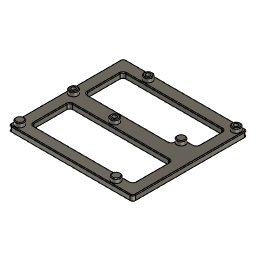
Manta-E3EZ_Mount (Autodesk Fusion 360 design; units mm, degrees)
Autodesk Fusion 360 part; units mm, degrees
sketch "Sketch1" plane through (0, 0, 0) normal (0, 0, 1) x (1, 0, 0)
  line L0 (0, 0) -> (120, 0)
  line L1 (120, 0) -> (120, 90.8)
  line L2 (120, 90.8) -> (0, 90.8)
  line L3 (0, 90.8) -> (0, 0)
  circle A0 centre (101.8, 77.23) radius 3
  circle A1 centre (39.65, 77.03) radius 3
  circle A2 centre (21.79, 42.05) radius 3
  circle A3 centre (53.59, 39.41) radius 3
  circle A4 centre (21.79, 4) radius 3
  circle A5 centre (90, 4) radius 3
  circle A6 centre (90, 50) radius 3
  circle A7 centre (21.79, 42.05) radius 1.45
  circle A8 centre (53.59, 39.41) radius 1.45
  circle A9 centre (39.65, 77.03) radius 1.45
  circle A10 centre (101.8, 77.23) radius 1.45
  line L4 (17.79, 0) -> (17.79, 90.8) construction
  line L5 (0, 81.23) -> (120, 81.23) construction
  line L6 (105.8, 90.8) -> (105.8, 0) construction
  line L7 (0, 35.41) -> (120, 35.41) construction
  line L8 (0, 46.05) -> (120, 46.05) construction
  line L9 (90, 90.8) -> (90, 0) construction
  line L10 (97.8, 90.8) -> (97.8, 0) construction
  line L11 (90, 53) -> (97.8, 53)
  line L12 (0, 73.03) -> (120, 73.03) construction
  line L13 (97.8, 73.03) -> (97.8, 53)
  line L14 (25.79, 90.8) -> (25.79, 0) construction
  line L15 (25.79, 73.03) -> (97.8, 73.03)
  line L16 (105.8, 81.23) -> (105.8, 0)
  line L17 (105.8, 81.23) -> (17.79, 81.23)
  line L18 (17.79, 81.23) -> (17.79, 0)
  line L19 (25.79, 73.03) -> (25.79, 46.05)
  line L20 (87, 90.8) -> (87, 0) construction
  line L21 (25.79, 8) -> (97.8, 8)
  line L22 (25.79, 8) -> (25.79, 35.41)
  line L23 (25.79, 35.41) -> (97.8, 35.41)
  line L24 (97.8, 35.41) -> (97.8, 8)
  line L25 (25.79, 46.05) -> (87, 46.05)
  line L26 (87, 46.05) -> (87, 50)
  dimension "d1" = 120
  dimension "d2" = 90.8
  dimension "d3" = 6
  dimension "d4" = 101.8
  dimension "d5" = 77.23
  dimension "d9" = 39.65
  dimension "d10" = 77.03
  dimension "d11" = 42.05
  dimension "d12" = 21.79
  dimension "d13" = 53.59
  dimension "d14" = 39.41
  dimension "d17" = 21.79
  dimension "d18" = 4
  dimension "d20" = 30
  dimension "d21" = 4
  dimension "d23" = 30
  dimension "d24" = 50
  dimension "d30" = 2.9
  dimension "d31" = 2.9
  dimension "d32" = 6
  dimension "d33" = 6
  dimension "d34" = 2.9
  dimension "d35" = 6
  dimension "d36" = 6
  dimension "d37" = 6
  dimension "d38" = 6
  dimension "d39" = 2.9
  dimension "d53" = 4
  dimension "d54" = 4
  dimension "d55" = 4
  dimension "d56" = 4
  dimension "d57" = 4
  dimension "d58" = 4
  dimension "d59" = 4
  dimension "d60" = 4
  dimension "d61" = 4
  constraint horizontal L0
  constraint vertical L1
  constraint horizontal L2
  constraint vertical L3
  constraint coincident L0.start L3.end
  constraint concentric A2 A7
  constraint concentric A3 A8
  constraint concentric A1 A9
  constraint concentric A0 A10
  constraint coincident L0 L4.start
  constraint coincident L2 L4.end
  constraint perpendicular L2 L4
  constraint coincident L3 L5.start
  constraint coincident L1 L5.end
  constraint perpendicular L1 L5
  constraint coincident L2 L6.start
  constraint coincident L0 L6.end
  constraint perpendicular L0 L6
  constraint coincident L3 L7.start
  constraint coincident L1 L7.end
  constraint perpendicular L1 L7
  constraint coincident L3 L8.start
  constraint coincident L1 L8.end
  constraint perpendicular L1 L8
  constraint coincident L2 L9.start
  constraint coincident L0 L9.end
  constraint perpendicular L0 L9
  constraint coincident A6.centre L9
  constraint coincident L2 L10.start
  constraint coincident L0 L10.end
  constraint perpendicular L0 L10
  constraint coincident A6 L11.start
  constraint coincident L9 L11.start
  constraint coincident L10 L11.end
  constraint tangent A6 L11
  constraint coincident L3 L12.start
  constraint coincident L1 L12.end
  constraint perpendicular L1 L12
  constraint coincident L12 L13.start
  constraint coincident L10 L13.start
  constraint coincident L2 L14.start
  constraint coincident L0 L14.end
  constraint perpendicular L0 L14
  constraint coincident L14 L15.start
  constraint coincident L12 L15.start
  constraint coincident L6 L16.start
  constraint coincident L5 L16.start
  constraint coincident L5 L17.end
  constraint coincident L4 L17.end
  constraint coincident L8 L19.end
  constraint coincident L14 L19.end
  constraint coincident L2 L20.start
  constraint coincident L0 L20.end
  constraint perpendicular L0 L20
  constraint tangent A6 L20
  constraint coincident L14 L21.start
  constraint coincident L10 L21.end
  constraint perpendicular L10 L21
  constraint coincident L14 L22.end
  constraint coincident L7 L22.end
  constraint coincident L10 L23.end
  constraint coincident L7 L23.end
  constraint coincident L8 L25.end
  constraint coincident L20 L25.end
  constraint coincident A6 L26.end
  constraint tangent A6 L26
  measures "d1" distance of L0.start L0.end
  measures "d2" distance of L0.start L2.end
  measures "d3" diameter of A0
  measures "d4" distance of L3 A0.centre
  measures "d5" distance of L0 A0.centre
  measures "d9" distance of L3 A1.centre
  measures "d10" distance of L0 A1.centre
  measures "d11" distance of L0 A2.centre
  measures "d12" distance of L3 A2.centre
  measures "d13" distance of L3 A3.centre
  measures "d14" distance of L0 A3.centre
  measures "d17" distance of L3 A4.centre
  measures "d18" distance of L0 A4.centre
  measures "d20" distance of L1 A5.centre
  measures "d21" distance of L0 A5.centre
  measures "d23" distance of L1 A6.centre
  measures "d24" distance of L0 A6.centre
  measures "d30" diameter of A10
  measures "d31" diameter of A7
  measures "d32" diameter of A2
  measures "d33" diameter of A1
  measures "d34" diameter of A9
  measures "d35" diameter of A4
  measures "d36" diameter of A5
  measures "d37" diameter of A6
  measures "d38" diameter of A3
  measures "d39" diameter of A8
  measures "d53" distance of A2.centre L4
  measures "d54" distance of A0.centre L5
  measures "d55" distance of A0.centre L6
  measures "d56" distance of A3.centre L7
  measures "d57" distance of A2.centre L8
  measures "d58" distance of A0.centre L10
  measures "d59" distance of A1.centre L12
  measures "d60" distance of A4.centre L14
  measures "d61" distance of A4.centre L21
extrude "Extrude4" add sketch "Sketch1" along normal blind 7 contours A0 | A1 | A2 | A3 | A4 | A5 | A6 makes body 1 at (90.8125, 52.8879, 2.3333) makes body 2 at (42.2847, 78.4648, 2.3333) makes body 3 at (50.6049, 39.1113, 4.6667) makes body 4 at (24.7751, 3.7013, 4.6667) makes body 5 at (102.7555, 80.0738, 4.6667) makes body 6 at (18.8049, 41.7513, 4.6667) makes body 7 at (90.9555, 6.8438, 4.6667)
extrude "Extrude6" add sketch "Sketch1" along normal blind 4 contours L0 L16 L17 L18 bodies 1 2 3 4 5 6 7
fillet "Fillet3" radius 2 13 edges at (97.8, 73.03, 2) (97.8, 35.41, 2) (17.79, 0, 2) (105.8, 0, 2) (17.79, 81.23, 2) (25.79, 73.03, 2) (105.8, 81.23, 2) (25.79, 35.41, 2) (25.79, 8, 2) (25.79, 46.05, 2) (97.8, 8, 2) (87, 46.05, 2) (97.8, 53, 2) on bodies 1
fillet "Fillet4" radius 0.5 27 edges at (87, 49.025, 4) (86.4142, 46.6358, 4) (56.395, 46.05, 4) (26.3758, 46.6358, 4) (25.79, 59.54, 4) (26.3758, 72.4442, 4) (61.795, 73.03, 4) (97.2142, 72.4442, 4) (97.8, 63.015, 4) (97.2142, 53.5858, 4) (92.9, 53, 4) (26.3758, 8.5858, 4) (61.795, 8, 4) (97.2142, 8.5858, 4) (97.8, 21.705, 4) (97.2142, 34.8242, 4) (61.795, 35.41, 4) (26.3758, 34.8242, 4) (25.79, 21.705, 4) (18.3758, 0.5858, 4) (61.795, 0, 4) (105.2142, 0.5858, 4) (105.8, 40.615, 4) (105.2142, 80.6442, 4) (61.795, 81.23, 4) (18.3758, 80.6442, 4) (17.79, 40.615, 4) on bodies 1
fillet "Fillet5" radius 0.5 7 edges at (87.203, 2.9152, 7) (18.993, 2.9152, 7) (18.993, 40.9652, 7) (50.793, 38.3252, 7) (87.203, 48.9152, 7) (99.003, 76.1452, 7) (36.853, 75.9452, 7) on bodies 1 2 3 4 5 6 7
chamfer "Chamfer1" distance 0.4 angle 45 28 edges at (61.795, 0, 0) (105.2142, 0.5858, 0) (105.8, 40.615, 0) (105.2142, 80.6442, 0) (61.795, 81.23, 0) (18.3758, 80.6442, 0) (17.79, 40.615, 0) (18.3758, 0.5858, 0) (56.395, 46.05, 0) (26.3758, 46.6358, 0) (25.79, 59.54, 0) (26.3758, 72.4442, 0) (61.795, 73.03, 0) (97.2142, 72.4442, 0) (97.8, 63.015, 0) (97.2142, 53.5858, 0) (92.9, 53, 0) (87.8787, 52.1213, 0) (87, 49.025, 0) (86.4142, 46.6358, 0) (61.795, 35.41, 0) (97.2142, 34.8242, 0) (97.8, 21.705, 0) (97.2142, 8.5858, 0) (61.795, 8, 0) (26.3758, 8.5858, 0) (25.79, 21.705, 0) (26.3758, 34.8242, 0) on bodies 1
equation "d3 = SupportPostDiameter"
equation "SupportPostDiameter = 6 mm"
equation "M3_PlasticThreads = 2.9 mm"
equation "SupportPostHeight = 7 mm"
equation "d30 = M3_PlasticThreads"
equation "d31 = M3_PlasticThreads"
equation "d32 = SupportPostDiameter"
equation "d33 = SupportPostDiameter"
equation "d34 = M3_PlasticThreads"
equation "d35 = SupportPostDiameter"
equation "d36 = SupportPostDiameter"
equation "d37 = SupportPostDiameter"
equation "d38 = SupportPostDiameter"
equation "d39 = M3_PlasticThreads"
equation "BaseHight = 4 mm"
equation "d53 = SupportPostDiameter / 2 + 1 mm"
equation "d54 = SupportPostDiameter / 2 + 1 mm"
equation "d55 = SupportPostDiameter / 2 + 1 mm"
equation "d56 = SupportPostDiameter / 2 + 1 mm"
equation "d57 = SupportPostDiameter / 2 + 1 mm"
equation "d58 = SupportPostDiameter / 2 + 1 mm"
equation "d59 = SupportPostDiameter / 2 + 1 mm"
equation "d60 = SupportPostDiameter / 2 + 1 mm"
equation "d61 = SupportPostDiameter / 2 + 1 mm"
equation "d62 = SupportPostHeight"
equation "d66 = BaseHight"
named bodies: "Manta-E3EZ_Mount"
